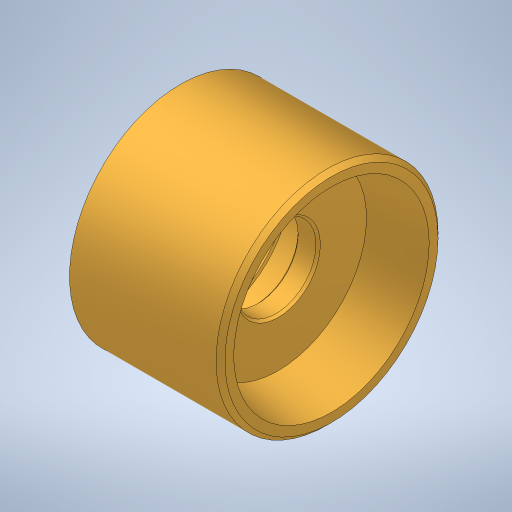
# Autodesk Inventor part: Flywheel
Saved by Autodesk Inventor 2023.2 (Build 272271000, 271)
## iProperties
Created: 2024-01-10
Part Number: Flywheel
Material: Brass, Soft Yellow
Document SubType Name: Modeling
Designer: Nathan Cai
Mass: 133.882 g
Surface Area: 92.12 cm^2
Volume: 15.8066 cm^3
Density: 8.47 g/cm^3
Appearance: Brass - Satin
Author: Nathan Cai
Autodesk Inventor part; units mm, degrees
ref_plane "YZ Plane" through (0, 0, 0) normal (1, 0, 0) x (0, 1, 0)
ref_plane "XZ Plane" through (0, 0, 0) normal (0, 1, 0) x (-1, 0, 0)
ref_plane "XY Plane" through (0, 0, 0) normal (0, 0, 1) x (1, 0, 0)
sketch "Sketch1" plane through (0, 0, 0) normal (0, 1, 0) x (-1, 0, 0)
  line L0 (0, 0) -> (5, 0)
  line L1 (5, 0) -> (5, -9)
  line L2 (5, -9) -> (0, -9)
  line L3 (0, -9) -> (0, 0)
  line L4 (5, 0) -> (17, 0)
  line L5 (17, 0) -> (17, -17.7)
  line L6 (17, -17.7) -> (5, -17.7)
  line L7 (5, -17.7) -> (5, 0)
  line L8 (0, 0) -> (-12, 0)
  line L9 (-12, 0) -> (-12, -25)
  line L10 (-12, -25) -> (0, -25)
  line L11 (0, -25) -> (0, 0)
  line L12 (-12, -22) -> (0, -19.8841)
  line L13 (-12, -28) -> (-12, 0)
  line L14 (-12, 0) -> (17, 0)
  line L15 (17, 0) -> (17, -25)
  line L16 (17, -25) -> (-12, -25)
  line L17 (-12, -25) -> (-12, 0)
  line L18 (-12, -25) -> (17, -19.8865)
  line L19 (17, -25) -> (22, -25)
  line L20 (22, -25) -> (22, -22)
  line L21 (22, -22) -> (17, -22)
  line L22 (17, -22) -> (17, -25)
  point P0 (5, -9)
  point P1 (0, -25)
  point P2 (17, -22)
  dimension "d0" = 5
  dimension "d1" = 9
  dimension "d2" = 12
  dimension "d3" = 17.7
  dimension "d6" = 12
  dimension "d7" = 25
  dimension "d8" = 80
  dimension "d9" = 22
  dimension "d35" = 5
  dimension "d36" = 22
  constraints: 46 end point, 11 parallel, 5 horizontal, 5 perpendicular, 5 point on line
  measures "d0" distance of L1.end L2.end
  measures "d1" distance of L0.end L1.end
  measures "d2" distance of L5.end L6.end
  measures "d3" distance of L4.end L5.end
  measures "d6" distance of L10.end L9.end
  measures "d7" distance of L9.end L8.end
  measures "d8" angle of L9 L12
  measures "d9" distance from line of L8 L12.start
  measures "d35" distance of L21.end L20.end
  measures "d36" distance between parallel lines of L8 L21
revolve "Revolution1" add sketch "Sketch1" angle 360 about axis through (0, 0, 0) along (-1, 0, 0) contours L2 L7 L6 L15 L18 L11 | L11 L18 L9 L12 | L18 L15 L16 L11 | L11 L10 L18 | L21 L20 L19 L15
chamfer "Chamfer2" distance 0.5 angle 45 2 edges at (-5, 0, 9) (0, 0, 9)
chamfer "Chamfer4" distance 1 angle 45 1 edges at (12, 0, 25)
chamfer "Chamfer5" distance 2 angle 45 1 edges at (-17, 0, 17.7)
body "Solid1"
